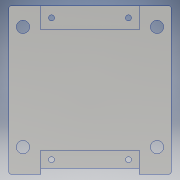
# Autodesk Inventor part: Part2
Saved by Autodesk Inventor 2018 (Build 220112000, 112)
## iProperties
Created: 2018-02-06
Part Number: Part2
Material: Aluminum 6061
Document SubType Name: Modeling
Designer: P136265
Density: 2.7 g/cm^3
Appearance: Aluminum - Flat
Author: P136265
Autodesk Inventor part; units mm, degrees
ref_plane "YZ Plane" through (0, 0, 0) normal (1, 0, 0) x (0, 1, 0)
ref_plane "XZ Plane" through (0, 0, 0) normal (0, 1, 0) x (-1, 0, 0)
ref_plane "XY Plane" through (0, 0, 0) normal (0, 0, 1) x (1, 0, 0)
sketch "Sketch1" plane through (0, 0, 0) normal (0, 1, 0) x (-1, 0, 0)
  line L0 (67.5, -70) -> (-67.5, -70)
  line L1 (-67.5, -70) -> (-67.5, 70)
  line L2 (-67.5, 70) -> (67.5, 70)
  line L3 (67.5, 70) -> (67.5, -70)
  line L4 (67.5, -70) -> (-67.5, 70) construction
  line L5 (-67.5, -70) -> (67.5, 70) construction
  circle A0 centre (-55.75, -52.5) radius 5.5
  circle A1 centre (55.75, -52.5) radius 5.5
  circle A2 centre (55.75, 47.5) radius 5.5
  circle A3 centre (-55.75, 47.5) radius 5.5
  line L6 (55.75, -52.5) -> (-55.75, -52.5) construction
  line L7 (55.75, 47.5) -> (-55.75, 47.5) construction
  line L8 (0, -70) -> (0, -52.5) construction
  line L9 (0, -52.5) -> (0, 0) construction
  line L10 (0, 0) -> (0, 47.5) construction
  line L11 (0, 70) -> (0, 47.5) construction
  point P0 (0, 0)
  point P1 (0, 0)
  point P2 (0, 0)
  dimension "d0" = 135
  dimension "d1" = 140
  dimension "d2" = 11
  dimension "d4" = 11
  dimension "d5" = 11
  dimension "d6" = 11
  dimension "d7" = 111.5
  dimension "d9" = 100
  dimension "d27" = 22.5
  constraints: 24 end point, 8 midpoint, 4 centre point, 3 horizontal, 2 collinear, 2 parallel, 2 vertical alignment, 1 coincident, 1 perpendicular
  measures "d0" distance of L1.end L2.end
  measures "d1" distance of L0.end L1.end
  measures "d2" diameter of A0
  measures "d4" diameter of A1
  measures "d5" diameter of A2
  measures "d6" diameter of A3
  measures "d7" distance of L6.end L6.start
  measures "d9" distance of L7.start L6.start
  measures "d27" distance from line of L2 L7.start
extrude "Extrusion1" add sketch "Sketch1" along normal blind 5
sketch "Sketch3" plane through (0, 5, 0) normal (0, 1, 0) x (1, 0, 0)
  circle A0 centre (55.75, -47.5) radius 5.5 construction
  circle A1 centre (-55.75, -47.5) radius 5.5 construction
  circle A2 centre (-55.75, 52.5) radius 5.5 construction
  circle A3 centre (55.75, 52.5) radius 5.5 construction
  line L0 (67.5, 70) -> (-67.5, 70) construction
  line L1 (-67.5, 70) -> (-67.5, -70) construction
  line L2 (-67.5, -70) -> (67.5, -70) construction
  line L3 (67.5, -70) -> (67.5, 70) construction
  line L4 (-41, -70) -> (41, -70)
  line L5 (-41, -50) -> (41, -50)
  line L6 (-41, -50) -> (-41, -70)
  line L7 (41, -50) -> (41, -70)
  line L8 (-67.5, -70) -> (67.5, -70) construction
  line L9 (-67.5, 70) -> (-67.5, -70) construction
  line L10 (-67.5, 0) -> (67.5, 0) construction
  line L11 (67.5, -70) -> (67.5, 70) construction
  line L12 (-41, 70) -> (41, 70)
  line L13 (-41, 50) -> (41, 50)
  line L14 (-41, 50) -> (-41, 70)
  line L15 (41, 50) -> (41, 70)
  point P0 (0, 0)
  point P1 (0, -70)
  point P2 (0, -70)
  point P3 (0, -70)
  dimension "d19" = 82
  dimension "d20" = 20
  constraints: 18 end point, 5 midpoint, 4 symmetric about line, 2 coincident, 2 parallel, 1 horizontal, 1 perpendicular
  measures "d19" distance of L4.start L4.end
  measures "d20" distance between parallel lines of L4 L5
extrude "Extrusion3" cut sketch "Sketch3" against normal blind 1
fillet "Fillet1" radius 2 4 edges at (67.5, 2.5, 70) (-67.5, 2.5, 70) (-67.5, 2.5, -70) (67.5, 2.5, -70)
sketch "Sketch4" plane through (0, 0, 0) normal (0, -1, 0) x (1, 0, 0)
  arc A0 (65.5, -70) -> (67.5, -68) centre (65.5, -68) ccw construction
  line L0 (67.5, -68) -> (67.5, 68) construction
  arc A1 (67.5, 68) -> (65.5, 70) centre (65.5, 68) ccw construction
  line L1 (65.5, 70) -> (-65.5, 70) construction
  arc A2 (-65.5, 70) -> (-67.5, 68) centre (-65.5, 68) ccw construction
  line L2 (-67.5, 68) -> (-67.5, -68) construction
  arc A3 (-67.5, -68) -> (-65.5, -70) centre (-65.5, -68) ccw construction
  line L3 (-65.5, -70) -> (65.5, -70) construction
  circle A4 centre (55.75, 47.5) radius 5.5 construction
  circle A5 centre (-55.75, 47.5) radius 5.5 construction
  circle A6 centre (-55.75, -52.5) radius 5.5 construction
  circle A7 centre (55.75, -52.5) radius 5.5 construction
  line L4 (-41, 70) -> (41, 70)
  line L5 (-41, 65) -> (41, 65)
  line L6 (-41, 70) -> (-41, 65)
  line L7 (41, 70) -> (41, 65)
  line L8 (65.5, 70) -> (-65.5, 70) construction
  point P0 (0, 0)
  point P1 (0, 70)
  point P2 (0, 70)
  point P3 (0, 70)
  dimension "d30" = 82
  dimension "d31" = 5
  constraints: 8 end point, 3 midpoint, 2 coincident, 2 parallel, 1 horizontal, 1 vertical
  measures "d30" distance of L4.start L4.end
  measures "d31" distance between parallel lines of L4 L5
extrude "Extrusion4" cut sketch "Sketch4" against normal up to next
sketch "Sketch6" plane through (0, 0, 0) normal (0, -1, 0) x (1, 0, 0)
  circle A0 centre (55.75, -52.5) radius 5.5 construction
  circle A1 centre (-55.75, -52.5) radius 5.5 construction
  circle A2 centre (-55.75, 47.5) radius 5.5 construction
  circle A3 centre (55.75, 47.5) radius 5.5 construction
  line L0 (41, 70) -> (41, 65) construction
  line L1 (41, 65) -> (-41, 65) construction
  line L2 (-41, 65) -> (-41, 70) construction
  line L3 (-41, 70) -> (-65.5, 70) construction
  arc A4 (-65.5, 70) -> (-67.5, 68) centre (-65.5, 68) ccw construction
  line L4 (-67.5, 68) -> (-67.5, -68) construction
  arc A5 (-67.5, -68) -> (-65.5, -70) centre (-65.5, -68) ccw construction
  line L5 (-65.5, -70) -> (65.5, -70) construction
  arc A6 (65.5, -70) -> (67.5, -68) centre (65.5, -68) ccw construction
  line L6 (67.5, -68) -> (67.5, 68) construction
  arc A7 (67.5, 68) -> (65.5, 70) centre (65.5, 68) ccw construction
  line L7 (65.5, 70) -> (41, 70) construction
  circle A8 centre (-32, 58) radius 3 construction
  circle A9 centre (32, 58) radius 3 construction
  circle A10 centre (-32, -60) radius 3 construction
  circle A11 centre (32, -60) radius 3 construction
  line L8 (-32, -60) -> (32, -60) construction
  line L9 (-32, 58) -> (32, 58) construction
  line L10 (-41, 50) -> (41, 50) construction
  line L11 (41, -50) -> (-41, -50) construction
  line L12 (-41, -50) -> (-41, -70) construction
  point P0 (0, 0)
  point P1 (0, 58)
  point P2 (0, 65)
  point P3 (0, -60)
  point P4 (0, -70)
  dimension "d51" = 6
  dimension "d52" = 6
  dimension "d53" = 6
  dimension "d54" = 6
  dimension "d55" = 8
  dimension "d56" = 9
  dimension "d57" = 10
  dimension "d59" = 9
  constraints: 4 centre point, 4 end point, 4 midpoint, 2 horizontal, 2 vertical alignment
  measures "d51" diameter of A8
  measures "d52" diameter of A9
  measures "d53" diameter of A10
  measures "d54" diameter of A11
  measures "d55" distance from line of L10 point (0, 58)
  measures "d56" horizontal distance of L10.start L9.start
  measures "d57" distance of point (0, -70) point (0, -60)
  measures "d59" distance from line of L12 L8.start
hole "Hole2" at (-32, 0, -60) at (32, 0, -60) at (-32, 0, 58) at (32, 0, 58) direction (0, 1, 0) diameter 5 end through all countersink diameter 11 countersink angle 90
body "Solid1"
